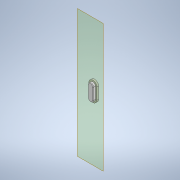
# Autodesk Inventor part: power_button
Saved by Autodesk Inventor 2022 (Build 260153000, 153)
## iProperties
Created: 2022-05-12
Part Number: power_button
Material: Generic
Document SubType Name: Modeling
Designer: simen
Density: 1 g/cm^3
Appearance: Default
Author: simen
## iProperties of the stored document power_button_3DPrint.ipt
Created: 2022-05-12
Part Number: power_button_3DPrint
Material: Generic
Document SubType Name: Modeling
Designer: simen
Density: 1 g/cm^3
Appearance: Default
Author: simen
Autodesk Inventor part; units mm, degrees
ref_plane "YZ Plane" through (0, 0, 0) normal (1, 0, 0) x (0, 1, 0)
ref_plane "XZ Plane" through (0, 0, 0) normal (0, 1, 0) x (-1, 0, 0)
ref_plane "XY Plane" through (0, 0, 0) normal (0, 0, 1) x (1, 0, 0)
ref_plane "Work Plane1" through (0, 1.5, -1.5) normal (0, 0, -1) x (-1, 0, 0)
sketch "Sketch1" plane through (0, 1.5, -1.5) normal (0, 0, -1) x (-1, 0, 0)
  line L0 (-0.5, 0.5) -> (-0.5, 101.5) projected
  line L1 (-20.5, 0.5) -> (-0.5, 0.5) projected
  line L2 (-20.5, 101.5) -> (-20.5, 0.5) projected
  line L3 (-0.5, 101.5) -> (-20.5, 101.5) projected
  line L4 (-15, 56) -> (-15, 46) projected
  arc A0 (-15, 46) -> (-10, 46) centre (-12.5, 46) ccw projected
  line L5 (-10, 46) -> (-10, 56) projected
  arc A1 (-10, 56) -> (-15, 56) centre (-12.5, 56) ccw projected
  arc A2 (-16, 46) -> (-9, 46) centre (-12.5, 46) ccw
  line L6 (-16, 46) -> (-16, 56)
  arc A3 (-9, 56) -> (-16, 56) centre (-12.5, 56) ccw
  line L7 (-9, 56) -> (-9, 46)
  point P0 (0, -1.5)
  dimension "d0" = 1
  constraints: 4 end point, 4 point on circle, 2 centre point, 3 other
  measures "d0" radial gap between concentric circles of A0 A2
extrude "Extrusion1" add sketch "Sketch1" along normal blind 1.5 contours A1 L5 A0 L4 | L6 A3 L7 A2
sketch "Sketch2" plane through (0, 1.5, -1.5) normal (0, 0, 1) x (1, 0, 0)
  line L0 (0.5, 0.5) -> (0.5, 101.5) projected
  line L1 (20.5, 0.5) -> (0.5, 0.5) projected
  line L2 (20.5, 101.5) -> (20.5, 0.5) projected
  line L3 (0.5, 101.5) -> (20.5, 101.5) projected
  line L4 (15, 56) -> (15, 46) projected
  arc A0 (10, 46) -> (15, 46) centre (12.5, 46) ccw projected
  line L5 (10, 46) -> (10, 56) projected
  arc A1 (15, 56) -> (10, 56) centre (12.5, 56) ccw projected
  line L6 (10.3, 56) -> (10.3, 46)
  arc A2 (10.3, 46) -> (14.7, 46) centre (12.5, 46) ccw
  line L7 (14.7, 46) -> (14.7, 56)
  arc A3 (14.7, 56) -> (10.3, 56) centre (12.5, 56) ccw
  point P0 (0, -1.5)
  dimension "d3" = 0.3
  constraints: 4 end point, 4 point on circle, 2 centre point, 3 other
  measures "d3" radial gap between concentric circles of A1 A3
extrude "Extrusion2" add sketch "Sketch2" along normal blind 2 contours A3 L7 A2 L6
fillet "Fillet1" radius 0.5 4 edges at (12.5, 59.7, 0.5) (10.3, 52.5, 0.5) (12.5, 45.3, 0.5) (14.7, 52.5, 0.5)
body "Solid1"
